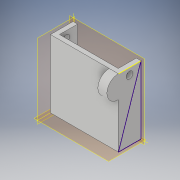
# Autodesk Inventor part: Scooop
Saved by Autodesk Inventor 2019 (Build 230136000, 136)
## iProperties
Created: 2019-05-08
Part Number: Scooop
Material: Generic
Document SubType Name: Modeling
Designer: codubois20
Density: 1 g/cm^3
Appearance: Default
Author: codubois20
Autodesk Inventor part; units mm, degrees
sketch "Sketch1" plane through (0, 0, 0) normal (0, 0, 1) x (1, 0, 0)
  line L0 (0, 0) -> (38.1, 0)
  line L1 (38.1, 0) -> (38.1, 38.1)
  line L2 (38.1, 38.1) -> (0, 38.1)
  line L3 (0, 38.1) -> (0, 0)
  dimension "d4" = 38.1
  dimension "d5" = 38.1
  constraints: 8 end point, 2 parallel, 1 horizontal, 1 perpendicular
  measures "d4" distance of L2.end L1.end
  measures "d5" distance of L1.end L0.end
extrude "Extrusion2" add sketch "Sketch1" along normal blind 12.7
sketch "Sketch4" plane through (0, 0, 0) normal (0, 0, -1) x (-1, 0, 0)
  line L0 (-38.1, 0) -> (-38.1, 38.1) projected
  line L1 (-35.56, 2.54) -> (-2.54, 2.54)
  line L2 (-2.54, 2.54) -> (-2.54, 35.56)
  line L3 (-38.1, 38.1) -> (0, 38.1) projected
  line L4 (-35.56, 35.56) -> (-35.56, 2.54)
  line L5 (-35.56, 35.56) -> (-35.56, 38.1)
  line L6 (-2.54, 35.56) -> (-2.54, 38.1)
  line L7 (-35.56, 38.1) -> (-2.54, 38.1)
  point P0 (0, 0)
  constraints: 12 end point, 3 perpendicular, 2 point on line, 1 horizontal, 1 vertical
extrude "Extrusion3" cut sketch "Sketch4" against normal blind 10.16
sketch "Sketch5" plane through (38.1, 0, 0) normal (1, 0, 0) x (0, 0, -1)
  line L0 (0, 38.1) -> (-12.7, 38.1) projected
  line L1 (-6.35, 38.1) -> (-6.35, 34.29) construction
  circle A0 centre (-6.35, 34.29) radius 1.905
  point P0 (0, 0)
  dimension "d13" = 3.81
  dimension "d14" = 3.81
  constraints: 2 end point, 1 centre point, 1 coincident, 1 midpoint, 1 vertical
  measures "d13" distance of L1.start L1.end
  measures "d14" diameter of A0
extrude "Extrusion4" cut sketch "Sketch5" against normal blind 50.8
sketch "Sketch6" plane through (38.1, 0, 0) normal (1, 0, 0) x (0, 0, -1)
  line L0 (-12.7, 38.1) -> (-12.7, 25.3897)
  line L1 (-12.7, 0) -> (-12.7, 38.1) projected
  line L2 (-12.7, 38.1) -> (-12.7, 25.3897)
  line L3 (-12.7, 31.7449) -> (-19.05, 31.7449) construction
  arc A0 (-12.7, 38.0949) -> (-19.05, 31.7449) centre (-12.7, 31.7449) ccw
  arc A1 (-19.05, 31.7449) -> (-12.7, 25.3949) centre (-12.7, 31.7449) ccw
  line L4 (-12.7, 25.3949) -> (-12.7, 38.0949)
  point P0 (0, 0)
  dimension "d17" = 6.35
  constraints: 8 end point, 6 point on circle, 3 coincident, 3 point on line, 2 centre point, 2 collinear, 1 concentric, 1 horizontal, 1 midpoint
  measures "d17" distance of L3.start L3.end
extrude "Extrusion5" add sketch "Sketch6" against normal blind 5.08
sketch "Sketch7" plane through (38.1, 0, 0) normal (1, 0, 0) x (0, 0, -1)
  line L0 (0, 38.1) -> (-12.7, 38.1) projected
  line L1 (0, 0) -> (-12.7, 0) projected
  line L2 (0, 38.1) -> (-12.7, 0)
  line L3 (-12.7, 0) -> (0, 0)
  line L4 (0, 0) -> (0, 38.1) projected
  line L5 (0, 38.1) -> (0, 0)
  line L6 (0, 38.1) -> (-12.7, 0)
  line L7 (-12.7, 0) -> (0, 0)
  line L8 (0, 0) -> (0, 38.1)
  constraints: 12 end point, 4 collinear
body "Solid2"
